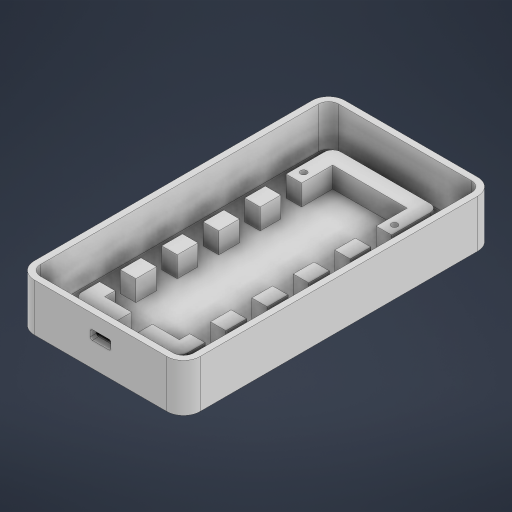
# Autodesk Inventor part: csing
Saved by Autodesk Inventor 2024 (Build 280153000, 153)
## iProperties
Created: 2025-06-11
Part Number: csing
Material: Generic
Document SubType Name: Modeling
Designer: ASUS
Density: 1 g/cm^3
Appearance: Default
Author: ASUS
Autodesk Inventor part; units mm, degrees
ref_plane "YZ Plane" through (0, 0, 0) normal (1, 0, 0) x (0, 1, 0)
ref_plane "XZ Plane" through (0, 0, 0) normal (0, 1, 0) x (-1, 0, 0)
ref_plane "XY Plane" through (0, 0, 0) normal (0, 0, 1) x (1, 0, 0)
sketch "Sketch1" plane through (0, 0, 0) normal (0, 1, 0) x (-1, 0, 0)
  line L0 (26.7027, -40.183) -> (-37.2973, -40.183)
  line L1 (-45.2973, -32.183) -> (-45.2973, 101.817)
  line L2 (-37.2973, 109.817) -> (26.7027, 109.817)
  line L3 (34.7027, 101.817) -> (34.7027, -32.183)
  arc A0 (26.7027, -40.183) -> (34.7027, -32.183) centre (26.7027, -32.183) ccw
  arc A1 (-45.2973, -32.183) -> (-37.2973, -40.183) centre (-37.2973, -32.183) ccw
  arc A2 (-37.2973, 109.817) -> (-45.2973, 101.817) centre (-37.2973, 101.817) ccw
  arc A3 (34.7027, 101.817) -> (26.7027, 109.817) centre (26.7027, 101.817) ccw
  point P0 (0, 0)
  point P1 (-45.2973, 109.817)
  point P2 (-45.2973, -40.183)
  point P3 (34.7027, 109.817)
  dimension "d0" = 80
  dimension "d1" = 150
  dimension "d2" = 8
  constraints: 8 end point, 8 point on circle, 8 tangent, 6 point on line, 4 centre point, 3 equal radius, 2 parallel, 1 horizontal, 1 perpendicular
  measures "d0" distance of point (-45.297, 109.817) point (34.703, 109.817)
  measures "d1" distance of point (-45.297, -40.183) point (-45.297, 109.817)
  measures "d2" radius of A0
extrude "Extrusion1" add sketch "Sketch1" along normal blind 3
sketch "Sketch2" plane through (0, 3, 0) normal (0, 1, 0) x (1, 0, 0)
  line L0 (-26.7027, 40.183) -> (37.2973, 40.183)
  line L1 (45.2973, 32.183) -> (45.2973, -101.817)
  line L2 (37.2973, -109.817) -> (-26.7027, -109.817)
  line L3 (-34.7027, -101.817) -> (-34.7027, 32.183)
  arc A0 (-26.7027, 40.183) -> (-34.7027, 32.183) centre (-26.7027, 32.183) ccw
  arc A1 (45.2973, 32.183) -> (37.2973, 40.183) centre (37.2973, 32.183) ccw
  arc A2 (37.2973, -109.817) -> (45.2973, -101.817) centre (37.2973, -101.817) ccw
  arc A3 (-34.7027, -101.817) -> (-26.7027, -109.817) centre (-26.7027, -101.817) ccw
  line L4 (37.2973, 37.183) -> (-26.7027, 37.183)
  arc A4 (-26.7027, 37.183) -> (-31.7027, 32.183) centre (-26.7027, 32.183) ccw
  line L5 (-31.7027, 32.183) -> (-31.7027, -101.817)
  arc A5 (-31.7027, -101.817) -> (-26.7027, -106.817) centre (-26.7027, -101.817) ccw
  line L6 (-26.7027, -106.817) -> (37.2973, -106.817)
  arc A6 (37.2973, -106.817) -> (42.2973, -101.817) centre (37.2973, -101.817) ccw
  line L7 (42.2973, -101.817) -> (42.2973, 32.183)
  arc A7 (42.2973, 32.183) -> (37.2973, 37.183) centre (37.2973, 32.183) ccw
  point P0 (0, 0)
  dimension "d5" = 8
  dimension "d6" = 3
  constraints: 16 end point, 16 point on circle, 8 centre point, 8 tangent, 4 parallel, 3 equal radius, 2 perpendicular, 1 horizontal, 7 other
  measures "d5" radius of A0
  measures "d6" distance between parallel lines of L0 L4
extrude "Extrusion2" add sketch "Sketch2" along normal blind 20
sketch "Sketch3" plane through (-26.7027, 0, 109.817) normal (0, 0, 1) x (1, 0, 0)
  line L0 (64, 0) -> (0, 0) projected
  line L1 (32, 0) -> (32, 14)
  line L2 (28, 16.25) -> (36, 16.25)
  line L3 (37, 15.25) -> (37, 12.75)
  line L4 (36, 11.75) -> (28, 11.75)
  line L5 (27, 12.75) -> (27, 15.25)
  line L6 (27, 16.25) -> (37, 11.75) construction
  line L7 (37, 16.25) -> (27, 11.75) construction
  arc A0 (28, 16.25) -> (27, 15.25) centre (28, 15.25) ccw
  arc A1 (37, 15.25) -> (36, 16.25) centre (36, 15.25) ccw
  arc A2 (36, 11.75) -> (37, 12.75) centre (36, 12.75) ccw
  arc A3 (27, 12.75) -> (28, 11.75) centre (28, 12.75) ccw
  point P0 (26.7027, 0)
  dimension "d9" = 14
  dimension "d10" = 10
  dimension "d11" = 4.5
  dimension "d14" = 1
  constraints: 14 end point, 8 point on circle, 8 point on line, 8 tangent, 4 centre point, 3 equal radius, 3 midpoint, 2 parallel, 1 horizontal, 1 perpendicular, 1 vertical
  measures "d9" distance of L1.start L1.end
  measures "d10" distance of L6.end L7.end
  measures "d11" distance of L7.start L6.end
  measures "d14" radius of A0
extrude "Extrusion3" cut sketch "Sketch3" against normal blind 3
sketch "Sketch4" plane through (0, 3, 0) normal (0, 1, 0) x (1, 0, 0)
  line L0 (37.2973, 37.183) -> (-26.7027, 37.183) projected
  line L1 (1.2973, -106.817) -> (9.2973, -106.817) projected
  line L2 (-31.7027, 32.183) -> (-31.7027, -101.817) projected
  line L3 (-12.7027, 20.183) -> (23.2973, 20.183)
  circle A0 centre (-16.6527, 10.133) radius 1.5
  circle A1 centre (27.2473, 10.133) radius 1.5
  circle A2 centre (-16.6527, -103.767) radius 1.5
  circle A3 centre (27.2473, -103.767) radius 1.5
  line L4 (26.7973, 27.683) -> (-16.2027, 27.683)
  arc A4 (-16.2027, 27.683) -> (-20.2027, 23.683) centre (-16.2027, 23.683) ccw
  arc A5 (30.7973, 23.683) -> (26.7973, 27.683) centre (26.7973, 23.683) ccw
  arc A6 (26.7973, -97.317) -> (30.7973, -93.317) centre (26.7973, -93.317) ccw
  arc A7 (-20.2027, -93.317) -> (-16.2027, -97.317) centre (-16.2027, -93.317) ccw
  arc A8 (-12.6907, -106.817) -> (-20.6147, -106.817) centre (-16.6527, -103.767) ccw
  line L5 (-20.6147, -106.817) -> (-12.6907, -106.817)
  line L6 (-26.7027, -109.817) -> (37.2973, -109.817) projected
  arc A9 (31.2093, -106.817) -> (23.2853, -106.817) centre (27.2473, -103.767) ccw
  line L7 (23.2853, -106.817) -> (31.2093, -106.817)
  line L8 (-20.2027, 5.183) -> (-12.7027, 5.183)
  line L9 (23.2973, 5.183) -> (30.7973, 5.183)
  line L10 (-20.2027, -4.817) -> (-12.7027, -4.817)
  line L11 (23.2973, -4.817) -> (30.7973, -4.817)
  line L12 (-20.2027, -14.817) -> (-12.7027, -14.817)
  line L13 (23.2973, -14.817) -> (30.7973, -14.817)
  line L14 (-20.2027, -24.817) -> (-12.7027, -24.817)
  line L15 (23.2973, -24.817) -> (30.7973, -24.817)
  line L16 (-20.2027, -34.817) -> (-12.7027, -34.817)
  line L17 (23.2973, -34.817) -> (30.7973, -34.817)
  line L18 (-20.2027, -44.817) -> (-12.7027, -44.817)
  line L19 (23.2973, -44.817) -> (30.7973, -44.817)
  line L20 (-20.2027, -54.817) -> (-12.7027, -54.817)
  line L21 (23.2973, -54.817) -> (30.7973, -54.817)
  line L22 (-20.2027, -64.817) -> (-12.7027, -64.817)
  line L23 (23.2973, -64.817) -> (30.7973, -64.817)
  line L24 (-20.2027, -74.817) -> (-12.7027, -74.817)
  line L25 (23.2973, -74.817) -> (30.7973, -74.817)
  line L26 (-20.2027, -84.817) -> (-12.7027, -84.817)
  line L27 (23.2973, -84.817) -> (30.7973, -84.817)
  line L28 (-12.7027, 5.183) -> (-12.7027, 20.183)
  line L29 (-20.2027, 23.683) -> (-20.2027, 5.183)
  line L30 (23.2973, 20.183) -> (23.2973, 5.183)
  line L31 (30.7973, 5.183) -> (30.7973, 23.683)
  line L32 (-12.7027, -89.817) -> (-12.7027, -84.817)
  line L33 (-20.2027, -84.817) -> (-20.2027, -93.317)
  line L34 (23.2973, -84.817) -> (23.2973, -89.817)
  line L35 (30.7973, -93.317) -> (30.7973, -84.817)
  line L36 (-12.7027, -74.817) -> (-12.7027, -64.817)
  line L37 (-20.2027, -64.817) -> (-20.2027, -74.817)
  line L38 (23.2973, -64.817) -> (23.2973, -74.817)
  line L39 (30.7973, -74.817) -> (30.7973, -64.817)
  line L40 (30.7973, -14.817) -> (30.7973, -4.817)
  line L41 (23.2973, -4.817) -> (23.2973, -14.817)
  line L42 (-12.7027, -14.817) -> (-12.7027, -4.817)
  line L43 (-20.2027, -4.817) -> (-20.2027, -14.817)
  line L44 (-20.2027, -24.817) -> (-20.2027, -34.817)
  line L45 (-20.2027, -44.817) -> (-20.2027, -54.817)
  line L46 (-12.7027, -54.817) -> (-12.7027, -44.817)
  line L47 (-12.7027, -34.817) -> (-12.7027, -24.817)
  line L48 (23.2973, -24.817) -> (23.2973, -34.817)
  line L49 (23.2973, -44.817) -> (23.2973, -54.817)
  line L50 (30.7973, -54.817) -> (30.7973, -44.817)
  line L51 (30.7973, -34.817) -> (30.7973, -24.817)
  line L52 (0.2973, -89.817) -> (0.2973, -97.317)
  line L53 (10.2973, -89.817) -> (10.2973, -97.317)
  line L54 (23.2973, -89.817) -> (10.2973, -89.817)
  line L55 (0.2973, -89.817) -> (-12.7027, -89.817)
  line L56 (-16.2027, -97.317) -> (0.2973, -97.317)
  line L57 (10.2973, -97.317) -> (26.7973, -97.317)
  point P0 (0, 0)
  dimension "d25" = 36
  dimension "d26" = 110
  dimension "d29" = 3
  dimension "d30" = 7.5
  dimension "d31" = 4
  dimension "d32" = 3.5
  dimension "d33" = 3.5
  constraints: 108 end point, 97 parallel, 30 tangent, 12 perpendicular, 12 point on circle, 10 centre point, 3 equal radius, 2 horizontal
  measures "d25" distance of L34.end L32.start
  measures "d26" distance of L3.end L34.end
  measures "d29" diameter of A0
  measures "d30" distance between parallel lines of L3 L4
  measures "d31" radius of A4
  measures "d32" radial gap between concentric circles of A2 A8
  measures "d33" radial gap between concentric circles of A3 A9
extrude "Extrusion4" add sketch "Sketch4" along normal blind 10
body "Solid1"
